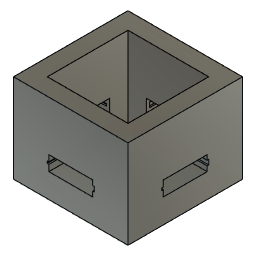
BTP_Rectangular_Final_Stopper (Autodesk Fusion 360 design; units mm, degrees)
Autodesk Fusion 360 part; units mm, degrees
sketch "Sketch1" plane through (0, 0, 0) normal (0, 0, 1) x (1, 0, 0)
  line L0 (-50, 50) -> (50, 50)
  line L1 (50, 50) -> (50, -50)
  line L2 (50, -50) -> (-50, -50)
  line L3 (-50, -50) -> (-50, 50)
  line L4 (71, 71) -> (71, -71)
  line L5 (71, -71) -> (-71, -71)
  line L6 (-71, -71) -> (-71, 71)
  line L7 (-71, 71) -> (71, 71)
  dimension "d1" = 100
  dimension "d2" = 100
  dimension "d5" = -21
  constraint horizontal L0
  constraint vertical L1
  constraint horizontal L2
  constraint vertical L3
  measures "d1" distance of L0.start L0.end
  measures "d2" distance of L0.start L2.end
extrude "Extrude1" add sketch "Sketch1" along normal blind 100
sketch "Sketch2" plane through (0, -71, 0) normal (0, -1, 0) x (1, 0, 0)
  line L0 (-71, 0) -> (71, 0)
  line L1 (71, 0) -> (71, 100)
  line L2 (71, 100) -> (-71, 100)
  line L3 (-71, 100) -> (-71, 0)
  line L4 (-28.65, 20) -> (28.65, 20)
  line L5 (28.65, 20) -> (28.65, 38.3)
  line L6 (28.65, 38.3) -> (-28.65, 38.3)
  line L7 (-28.65, 38.3) -> (-28.65, 20)
  dimension "d8" = 57.3
  dimension "d9" = 18.3
  constraint horizontal L4
  constraint vertical L5
  constraint horizontal L6
  constraint vertical L7
  measures "d8" distance of L4.start L4.end
  measures "d9" distance of L4.start L6.end
sketch "Sketch3" plane through (71, 0, 0) normal (1, 0, 0) x (0, 1, 0)
  line L0 (-71, 0) -> (71, 0)
  line L1 (71, 0) -> (71, 100)
  line L2 (71, 100) -> (-71, 100)
  line L3 (-71, 100) -> (-71, 0)
  line L4 (-28.65, 19.9999) -> (28.65, 19.9999)
  line L5 (28.65, 19.9999) -> (28.65, 38.2999)
  line L6 (28.65, 38.2999) -> (-28.65, 38.2999)
  line L7 (-28.65, 38.2999) -> (-28.65, 19.9999)
  dimension "d11" = 57.3
  dimension "d12" = 18.3
  constraint horizontal L4
  constraint vertical L5
  constraint horizontal L6
  constraint vertical L7
  measures "d11" distance of L4.start L4.end
  measures "d12" distance of L4.start L6.end
sketch "Sketch4" plane through (0, 71, 0) normal (0, 1, 0) x (-1, 0, 0)
  line L0 (-71, 0) -> (71, 0)
  line L1 (71, 0) -> (71, 100)
  line L2 (71, 100) -> (-71, 100)
  line L3 (-71, 100) -> (-71, 0)
sketch "Sketch5" plane through (0, -71, 0) normal (0, -1, 0) x (1, 0, 0)
sketch "Sketch6" plane through (0, 71, 0) normal (0, 1, 0) x (-1, 0, 0)
  line L0 (-70, 20) -> (-27.65, 20)
  line L1 (-27.65, 20) -> (29.65, 20)
  line L2 (29.65, 20) -> (29.65, 38.3)
  line L3 (29.65, 38.3) -> (-27.65, 38.3)
  line L4 (-27.65, 38.3) -> (-27.65, 20)
  dimension "d13" = 42.35
  dimension "d14" = 57.3
  dimension "d15" = 18.3
  constraint horizontal L0
  constraint horizontal L1
  constraint vertical L2
  constraint horizontal L3
  constraint vertical L4
  measures "d13" distance of L0.start L0.end
  measures "d14" distance of L0.end L1.end
  measures "d15" distance of L0.end L3.end
sketch "Sketch7" plane through (-71, 0, 0) normal (-1, 0, 0) x (0, -1, 0)
  line L0 (-71, 0) -> (71, 0)
  line L1 (71, 0) -> (71, 100)
  line L2 (71, 100) -> (-71, 100)
  line L3 (-71, 100) -> (-71, 0)
  line L4 (-28.65, 19.9999) -> (28.65, 19.9999)
  line L5 (28.65, 19.9999) -> (28.65, 38.2999)
  line L6 (28.65, 38.2999) -> (-28.65, 38.2999)
  line L7 (-28.65, 38.2999) -> (-28.65, 19.9999)
  dimension "d17" = 57.3
  dimension "d18" = 18.3
  constraint horizontal L4
  constraint vertical L5
  constraint horizontal L6
  constraint vertical L7
  measures "d17" distance of L4.start L4.end
  measures "d18" distance of L4.start L6.end
sketch "Sketch8" plane through (71, 0, 0) normal (1, 0, 0) x (0, 1, 0)
sketch "Sketch9" plane through (0, -71, 0) normal (0, -1, 0) x (1, 0, 0)
sketch "Sketch10" plane through (0, 71, 0) normal (0, 1, 0) x (-1, 0, 0)
sketch "Sketch11" plane through (71, 0, 0) normal (1, 0, 0) x (0, 1, 0)
extrude "Extrude2" cut sketch "Sketch2" against normal blind 21 contours L4 L5 L6 L7
extrude "Extrude3" cut sketch "Sketch3" against normal blind 21 contours L4 L5 L6 L7
extrude "Extrude4" cut sketch "Sketch6" against normal blind 21
extrude "Extrude5" cut sketch "Sketch7" against normal blind 21 contours L4 L5 L6 L7
sketch "Sketch12" plane through (0, 0, 0) normal (0, 0, 1) x (1, 0, 0)
  line L0 (71, 71) -> (-71, 71)
  line L1 (-71, 71) -> (-71, -71)
  line L2 (-71, -71) -> (71, -71)
  line L3 (71, -71) -> (71, 71)
  constraint horizontal L0
  constraint vertical L1
  constraint horizontal L2
  constraint vertical L3
extrude "Extrude6" add sketch "Sketch12" against normal blind 10
sketch "Sketch13" plane through (0, 0, 0) normal (0, 0, 1) x (-1, 0, 0)
  line L0 (-50, 50) -> (-50, -50)
  line L1 (-50, -50) -> (50, -50)
  line L2 (50, -50) -> (50, 50)
  line L3 (50, 50) -> (-50, 50)
move_body "Move1" bodies 1 to x (1, 0, 0) y (0, 1, 0) z (0, 0, 1) at (0, 0, 10)
extrude "Extrude7" add 1 faces at (-64, 28.65, 42.1999) along direction (0, -1, 0) blind 1.45
extrude "Extrude8" add 1 faces at (-64, -28.65, 36.0999) along direction (0, 1, 0) blind 1.45
sketch "Sketch14" plane through (-71, 0, 0) normal (-1, 0, 0) x (0, -1, 0)
  line L0 (27.2, 29.9999) -> (-27.2, 29.9999)
  line L1 (-27.2, 29.9999) -> (-27.2, 48.2999)
  line L2 (-27.2, 48.2999) -> (27.2, 48.2999)
  line L3 (27.2, 48.2999) -> (27.2, 29.9999)
  line L4 (71, 0) -> (71, 110)
  line L5 (71, 110) -> (-71, 110)
  line L6 (-71, 110) -> (-71, 0)
  line L7 (-71, 0) -> (71, 0)
  line L8 (-27.2, 40.5499) -> (-29.2, 40.5499)
  line L9 (-29.2, 40.5499) -> (-29.2, 37.8499)
  line L10 (-29.2, 37.8499) -> (-27.2, 37.8499)
  line L11 (-27.2, 37.8499) -> (-27.2, 40.5499)
  dimension "d34" = 2
  dimension "d35" = 2.7
  constraint perpendicular L8 L9
  constraint coincident L1 L10.end
  constraint perpendicular L1 L10
  measures "d34" distance of L8.start L8.end
  measures "d35" distance of L8.end L9.end
extrude "Extrude9" cut sketch "Sketch14" against normal blind 21.3 contours L1 L8 L9 L10 L11
sketch "Sketch15" plane through (-71, 0, 0) normal (-1, 0, 0) x (0, -1, 0)
  line L0 (-29.2, 40.5499) -> (-27.2, 40.5499)
  line L1 (-27.2, 40.5499) -> (-27.2, 48.2999)
  line L2 (-27.2, 48.2999) -> (27.2, 48.2999)
  line L3 (27.2, 48.2999) -> (27.2, 29.9999)
  line L4 (27.2, 29.9999) -> (-27.2, 29.9999)
  line L5 (-27.2, 29.9999) -> (-27.2, 37.8499)
  line L6 (-27.2, 37.8499) -> (-29.2, 37.8499)
  line L7 (-29.2, 37.8499) -> (-29.2, 40.5499)
  line L8 (71, 0) -> (71, 110)
  line L9 (71, 110) -> (-71, 110)
  line L10 (-71, 110) -> (-71, 0)
  line L11 (-71, 0) -> (71, 0)
  line L12 (27.2, 42.1999) -> (29.2, 42.1999)
  line L13 (29.2, 42.1999) -> (29.2, 36.1999)
  line L14 (29.2, 36.1999) -> (27.2, 36.1999)
  line L15 (27.2, 36.1999) -> (27.2, 42.1999)
  constraint perpendicular L3 L12
  constraint perpendicular L12 L13
  constraint coincident L3 L14.end
  constraint perpendicular L13 L14
extrude "Extrude10" cut sketch "Sketch15" against normal blind 21.3 contours L3 L12 L13 L14 L15
extrude "Extrude11" add 1 faces at (-28.65, -64, 42.2) along direction (1, 0, 0) blind 1.45
extrude "Extrude12" add 1 faces at (28.65, -64, 36.1) along direction (-1, 0, 0) blind 1.45
sketch "Sketch16" plane through (0, -71, 0) normal (0, -1, 0) x (1, 0, 0)
  line L0 (27.2, 30) -> (-27.2, 30)
  line L1 (-27.2, 30) -> (-27.2, 48.3)
  line L2 (-27.2, 48.3) -> (27.2, 48.3)
  line L3 (27.2, 48.3) -> (27.2, 30)
  line L4 (71, 0) -> (71, 110)
  line L5 (71, 110) -> (-71, 110)
  line L6 (-71, 110) -> (-71, 0)
  line L7 (-71, 0) -> (71, 0)
  line L8 (-27.2, 40.55) -> (-29.2, 40.55)
  line L9 (-29.2, 40.55) -> (-29.2, 37.85)
  line L10 (-29.2, 37.85) -> (-27.2, 37.85)
  line L11 (-27.2, 40.55) -> (-27.2, 37.85)
  constraint perpendicular L8 L9
  constraint perpendicular L1 L10
extrude "Extrude13" cut sketch "Sketch16" against normal blind 21.3 contours L1 L8 L9 L10 L11
sketch "Sketch17" plane through (0, -71, 0) normal (0, -1, 0) x (1, 0, 0)
  line L0 (-29.2, 40.55) -> (-27.2, 40.55)
  line L1 (-27.2, 40.55) -> (-27.2, 48.3)
  line L2 (-27.2, 48.3) -> (27.2, 48.3)
  line L3 (27.2, 48.3) -> (27.2, 30)
  line L4 (27.2, 30) -> (-27.2, 30)
  line L5 (-27.2, 30) -> (-27.2, 37.85)
  line L6 (-27.2, 37.85) -> (-29.2, 37.85)
  line L7 (-29.2, 37.85) -> (-29.2, 40.55)
  line L8 (71, 0) -> (71, 110)
  line L9 (71, 110) -> (-71, 110)
  line L10 (-71, 110) -> (-71, 0)
  line L11 (-71, 0) -> (71, 0)
  line L12 (27.2, 48.3) -> (27.2, 42.2)
  line L13 (27.2, 42.2) -> (29.2, 42.2)
  line L14 (29.2, 42.2) -> (29.2, 36.2)
  line L15 (29.2, 36.2) -> (27.2, 36.2)
  line L16 (27.2, 36.2) -> (27.2, 42.2)
  constraint coincident L2.end L3.start
  constraint perpendicular L2 L12
  constraint perpendicular L12 L13
  constraint perpendicular L13 L14
  constraint coincident L3 L15.end
  constraint perpendicular L3 L15
extrude "Extrude14" cut sketch "Sketch17" against normal blind 21 contours L3 L13 L14 L15 L16
extrude "Extrude15" add 1 faces at (64, -28.65, 42.1999) along direction (0, 1, 0) blind 1.45
extrude "Extrude16" add 1 faces at (64, 28.65, 36.0999) along direction (0, -1, 0) blind 1.45
sketch "Sketch18" plane through (71, 0, 0) normal (1, 0, 0) x (0, 1, 0)
  line L0 (27.2, 29.9999) -> (-27.2, 29.9999)
  line L1 (-27.2, 29.9999) -> (-27.2, 48.2999)
  line L2 (-27.2, 48.2999) -> (27.2, 48.2999)
  line L3 (27.2, 48.2999) -> (27.2, 29.9999)
  line L4 (71, 0) -> (71, 110)
  line L5 (71, 110) -> (-71, 110)
  line L6 (-71, 110) -> (-71, 0)
  line L7 (-71, 0) -> (71, 0)
  line L8 (-27.2, 40.5499) -> (-29.2, 40.5499)
  line L9 (-29.2, 40.5499) -> (-29.2, 37.8499)
  line L10 (-29.2, 37.8499) -> (-27.2, 37.8499)
  line L11 (-27.2, 37.8499) -> (-27.2, 40.5499)
  constraint perpendicular L1 L8
  constraint perpendicular L8 L9
  constraint coincident L1 L10.end
  constraint perpendicular L1 L10
extrude "Extrude17" cut sketch "Sketch18" against normal blind 21.3 contours L1 L8 L9 L10 L11
sketch "Sketch19" plane through (71, 0, 0) normal (1, 0, 0) x (0, 1, 0)
  line L0 (-29.2, 40.5499) -> (-27.2, 40.5499)
  line L1 (-27.2, 40.5499) -> (-27.2, 48.2999)
  line L2 (-27.2, 48.2999) -> (27.2, 48.2999)
  line L3 (27.2, 48.2999) -> (27.2, 29.9999)
  line L4 (27.2, 29.9999) -> (-27.2, 29.9999)
  line L5 (-27.2, 29.9999) -> (-27.2, 37.8499)
  line L6 (-27.2, 37.8499) -> (-29.2, 37.8499)
  line L7 (-29.2, 37.8499) -> (-29.2, 40.5499)
  line L8 (71, 0) -> (71, 110)
  line L9 (71, 110) -> (-71, 110)
  line L10 (-71, 110) -> (-71, 0)
  line L11 (-71, 0) -> (71, 0)
  line L12 (27.2, 48.2999) -> (27.2, 42.1999)
  line L13 (27.2, 42.1999) -> (29.2, 42.1999)
  line L14 (29.2, 42.7725) -> (29.2, 36.7725)
  line L15 (29.2, 36.7725) -> (27.2, 36.7725)
  line L16 (27.2, 36.7725) -> (27.2, 42.7725)
  constraint coincident L2.end L3.start
  constraint perpendicular L2 L12
  constraint perpendicular L3 L13
  constraint perpendicular L13 L14
  constraint coincident L3 L15.end
  constraint perpendicular L3 L15
  constraint perpendicular L15 L16
extrude "Extrude18" cut sketch "Sketch19" against normal blind 21.3 contours L3 L13 L14 L15 L16
sketch "Sketch20" plane through (0, 71, 0) normal (0, 1, 0) x (-1, 0, 0)
extrude "Extrude19" add 1 faces at (27.65, 64, 42.2) along direction (-1, 0, 0) blind 1.45
extrude "Extrude20" add 1 faces at (-29.65, 64, 36.1) along direction (1, 0, 0) blind 1.45
sketch "Sketch21" plane through (0, 71, 0) normal (0, 1, 0) x (-1, 0, 0)
sketch "Sketch22" plane through (-71, 0, 0) normal (-1, 0, 0) x (0, -1, 0)
  line L0 (29.2, 36.1999) -> (27.2, 36.1999)
  line L1 (27.2, 36.1999) -> (27.2, 29.9999)
  line L2 (27.2, 29.9999) -> (-27.2, 29.9999)
  line L3 (-27.2, 29.9999) -> (-27.2, 37.8499)
  line L4 (-27.2, 37.8499) -> (-29.2, 37.8499)
  line L5 (-29.2, 37.8499) -> (-29.2, 40.5499)
  line L6 (-29.2, 40.5499) -> (-27.2, 40.5499)
  line L7 (-27.2, 40.5499) -> (-27.2, 48.2999)
  line L8 (-27.2, 48.2999) -> (27.2, 48.2999)
  line L9 (27.2, 48.2999) -> (27.2, 42.1999)
  line L10 (27.2, 42.1999) -> (29.2, 42.1999)
  line L11 (29.2, 42.1999) -> (29.2, 36.1999)
  line L12 (71, 0) -> (71, 110)
  line L13 (71, 110) -> (-71, 110)
  line L14 (-71, 110) -> (-71, 0)
  line L15 (-71, 0) -> (71, 0)
extrude "Extrude21" add 1 faces at (-28.2, 64, 36.1) along direction (1, 0, 0) blind 1.02
extrude "Extrude22" cut 1 faces at (26.2, 64, 42.2) along direction (1, 0, 0) blind 1.02
sketch "Sketch23" plane through (0, 71, 0) normal (0, 1, 0) x (-1, 0, 0)
sketch "Sketch24" plane through (0, 71, 0) normal (0, 1, 0) x (-1, 0, 0)
  line L0 (-27.22, 40.55) -> (-29.22, 40.55)
  line L1 (-29.22, 40.55) -> (-29.22, 37.85)
  line L2 (-29.22, 37.85) -> (-27.22, 37.85)
  line L3 (-27.22, 37.85) -> (-27.22, 40.55)
  constraint perpendicular L0 L1
  constraint perpendicular L1 L2
extrude "Extrude23" cut sketch "Sketch24" against normal blind 21.3
sketch "Sketch25" plane through (0, 71, 0) normal (0, 1, 0) x (-1, 0, 0)
  line L0 (27.18, 42.2) -> (29.18, 42.2)
  line L1 (29.18, 42.2) -> (29.18, 36.2)
  line L2 (29.18, 36.2) -> (27.18, 36.2)
  line L3 (27.18, 42.2) -> (27.18, 36.2)
  constraint perpendicular L0 L1
  constraint perpendicular L1 L2
extrude "Extrude24" cut sketch "Sketch25" against normal blind 21.3
sketch "Sketch26" plane through (71, 0, 0) normal (1, 0, 0) x (0, 1, 0)
  line L0 (29.2, 36.7725) -> (27.2, 36.7725)
  line L1 (27.2, 36.7725) -> (27.2, 29.9999)
  line L2 (27.2, 29.9999) -> (-27.2, 29.9999)
  line L3 (-27.2, 29.9999) -> (-27.2, 37.8499)
  line L4 (-27.2, 37.8499) -> (-29.2, 37.8499)
  line L5 (-29.2, 37.8499) -> (-29.2, 40.5499)
  line L6 (-29.2, 40.5499) -> (-27.2, 40.5499)
  line L7 (-27.2, 40.5499) -> (-27.2, 48.2999)
  line L8 (-27.2, 48.2999) -> (27.2, 48.2999)
  line L9 (27.2, 48.2999) -> (27.2, 42.1999)
  line L10 (27.2, 42.1999) -> (29.2, 42.1999)
  line L11 (29.2, 42.1999) -> (29.2, 36.7725)
  line L12 (71, 0) -> (71, 110)
  line L13 (71, 110) -> (-71, 110)
  line L14 (-71, 110) -> (-71, 0)
  line L15 (-71, 0) -> (71, 0)
sketch "Sketch27" plane through (71, 0, 0) normal (1, 0, 0) x (0, 1, 0)
sketch "Sketch28" plane through (29.2, 0, 0) normal (-1, 0, 0) x (0, -1, 0)
  line L0 (71, 36.2) -> (71, 42.2)
  line L1 (71, 42.2) -> (50, 42.2)
  line L2 (50, 42.2) -> (50, 36.2)
  line L3 (50, 36.2) -> (71, 36.2)
  line L4 (50, 42.2) -> (55, 42.2)
  line L5 (55, 42.2) -> (55, 36.2)
  line L6 (55, 36.2) -> (50, 36.2)
  line L7 (50, 36.2) -> (50, 42.2)
  dimension "d93" = 5
  constraint horizontal L4
  constraint vertical L5
  constraint horizontal L6
  constraint vertical L7
  constraint coincident L1.end L2.start
  measures "d93" distance of L1.end L4.end
extrude "Extrude25" add sketch "Sketch28" along normal blind 2 contours L1 L2 L3 L4 L5 L6 L7
extrude "Extrude26" cut 1 faces at (28.5333, -55, 40.2) along direction (0, 1, 0) blind 1
sketch "Sketch29" plane through (0, -71, 0) normal (0, -1, 0) x (1, 0, 0)
  line L0 (29.2, 36.2) -> (27.2, 36.2)
  line L1 (27.2, 36.2) -> (27.2, 30)
  line L2 (27.2, 30) -> (-27.2, 30)
  line L3 (-27.2, 30) -> (-27.2, 37.85)
  line L4 (-27.2, 37.85) -> (-29.2, 37.85)
  line L5 (-29.2, 37.85) -> (-29.2, 40.55)
  line L6 (-29.2, 40.55) -> (-27.2, 40.55)
  line L7 (-27.2, 40.55) -> (-27.2, 48.3)
  line L8 (-27.2, 48.3) -> (27.2, 48.3)
  line L9 (27.2, 48.3) -> (27.2, 42.2)
  line L10 (27.2, 42.2) -> (29.2, 42.2)
  line L11 (29.2, 42.2) -> (29.2, 36.2)
  line L12 (71, 0) -> (71, 110)
  line L13 (71, 110) -> (-71, 110)
  line L14 (-71, 110) -> (-71, 0)
  line L15 (-71, 0) -> (71, 0)
sketch "Sketch30" plane through (71, 0, 0) normal (1, 0, 0) x (0, 1, 0)
sketch "Sketch31" plane through (-29.2, 0, 0) normal (1, 0, 0) x (0, 1, 0)
  line L0 (-50, 37.85) -> (-50, 40.55)
  line L1 (-50, 40.55) -> (-71, 40.55)
  line L2 (-71, 40.55) -> (-71, 37.85)
  line L3 (-71, 37.85) -> (-50, 37.85)
  line L4 (-50, 40.55) -> (-54, 40.55)
  line L5 (-54, 40.55) -> (-54, 37.85)
  line L6 (-54, 37.85) -> (-50, 37.85)
  line L7 (-50, 37.85) -> (-50, 40.55)
  dimension "d98" = 4
  constraint horizontal L4
  constraint vertical L5
  constraint horizontal L6
  constraint vertical L7
  constraint coincident L0.end L1.start
  measures "d98" distance of L0.end L4.end
extrude "Extrude27" add sketch "Sketch31" along normal blind 2 contours L0 L1 L3 L4 L5 L6 L7
sketch "Sketch32" plane through (-29.18, 0, 0) normal (1, 0, 0) x (0, 1, 0)
  line L0 (50, 42.2) -> (50, 36.2)
  line L1 (50, 36.2) -> (71, 36.2)
  line L2 (71, 36.2) -> (71, 42.2)
  line L3 (71, 42.2) -> (50, 42.2)
  line L4 (50, 42.2) -> (54, 42.2)
  line L5 (54, 42.2) -> (54, 36.2)
  line L6 (54, 36.2) -> (50, 36.2)
  line L7 (50, 36.2) -> (50, 42.2)
  dimension "d101" = 4
  constraint horizontal L4
  constraint vertical L5
  constraint horizontal L6
  constraint vertical L7
  constraint coincident L0.start L3.end
  measures "d101" distance of L0.start L4.end
extrude "Extrude28" add sketch "Sketch32" along normal blind 2 contours L0 L1 L3 L4 L5 L6 L7
sketch "Sketch33" plane through (29.22, 0, 0) normal (-1, 0, 0) x (0, -1, 0)
  line L0 (-50, 37.85) -> (-50, 40.55)
  line L1 (-50, 40.55) -> (-71, 40.55)
  line L2 (-71, 40.55) -> (-71, 37.85)
  line L3 (-71, 37.85) -> (-50, 37.85)
  line L4 (-50, 40.55) -> (-54, 40.55)
  line L5 (-54, 40.55) -> (-54, 37.85)
  line L6 (-54, 37.85) -> (-50, 37.85)
  line L7 (-50, 37.85) -> (-50, 40.55)
  dimension "d104" = 4
  constraint horizontal L4
  constraint vertical L5
  constraint horizontal L6
  constraint vertical L7
  constraint coincident L0.end L1.start
  measures "d104" distance of L0.end L4.end
extrude "Extrude29" add sketch "Sketch33" along normal blind 2 contours L0 L1 L3 L4 L5 L6 L7
sketch "Sketch34" plane through (0, -29.2, 0) normal (0, 1, 0) x (-1, 0, 0)
  line L0 (50, 42.1999) -> (50, 36.1999)
  line L1 (50, 36.1999) -> (71, 36.1999)
  line L2 (71, 36.1999) -> (71, 42.1999)
  line L3 (71, 42.1999) -> (50, 42.1999)
  line L4 (50, 42.1999) -> (54, 42.1999)
  line L5 (54, 42.1999) -> (54, 36.1999)
  line L6 (54, 36.1999) -> (50, 36.1999)
  line L7 (50, 36.1999) -> (50, 42.1999)
  dimension "d107" = 4
  constraint horizontal L4
  constraint vertical L5
  constraint horizontal L6
  constraint vertical L7
  constraint coincident L0.start L3.end
  measures "d107" distance of L0.start L4.end
extrude "Extrude30" add sketch "Sketch34" along normal blind 2 contours L0 L1 L3 L4 L5 L6 L7
sketch "Sketch35" plane through (0, 29.2, 0) normal (0, -1, 0) x (1, 0, 0)
  line L0 (-50, 37.8499) -> (-50, 40.5499)
  line L1 (-50, 40.5499) -> (-71, 40.5499)
  line L2 (-71, 40.5499) -> (-71, 37.8499)
  line L3 (-71, 37.8499) -> (-50, 37.8499)
  line L4 (-50, 40.5499) -> (-54, 40.5499)
  line L5 (-54, 40.5499) -> (-54, 37.8499)
  line L6 (-54, 37.8499) -> (-50, 37.8499)
  line L7 (-50, 37.8499) -> (-50, 40.5499)
  dimension "d110" = 4
  constraint horizontal L4
  constraint vertical L5
  constraint horizontal L6
  constraint vertical L7
  constraint coincident L0.end L1.start
  measures "d110" distance of L0.end L4.end
extrude "Extrude31" add sketch "Sketch35" along normal blind 2 contours L0 L1 L3 L4 L5 L6 L7
sketch "Sketch36" plane through (0, 29.2, 0) normal (0, -1, 0) x (1, 0, 0)
  line L0 (50, 42.1999) -> (50, 36.7725)
  line L1 (50, 36.7725) -> (71, 36.7725)
  line L2 (71, 36.7725) -> (71, 42.1999)
  line L3 (71, 42.1999) -> (50, 42.1999)
sketch "Sketch37" plane through (0, -29.2, 0) normal (0, 1, 0) x (-1, 0, 0)
  line L0 (-50, 37.8499) -> (-50, 40.5499)
  line L1 (-50, 40.5499) -> (-71, 40.5499)
  line L2 (-71, 40.5499) -> (-71, 37.8499)
  line L3 (-71, 37.8499) -> (-50, 37.8499)
  line L4 (-50, 40.5499) -> (-54, 40.5499)
  line L5 (-54, 40.5499) -> (-54, 37.8499)
  line L6 (-54, 37.8499) -> (-50, 37.8499)
  line L7 (-50, 37.8499) -> (-50, 40.5499)
  dimension "d113" = 4
  constraint horizontal L4
  constraint vertical L5
  constraint horizontal L6
  constraint vertical L7
  constraint coincident L0.end L1.start
  measures "d113" distance of L0.end L4.end
extrude "Extrude32" add sketch "Sketch37" along normal blind 2 contours L0 L1 L3 L4 L5 L6 L7
extrude "Extrude33" cut 1 faces at (64, 28.5333, 36.7725) along direction (0, 0, -1) blind 0.573
sketch "Sketch38" plane through (0, 29.2, 0) normal (0, -1, 0) x (1, 0, 0)
